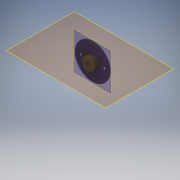
# Autodesk Inventor part: capot_inf
Saved by Autodesk Inventor 2018 (Build 220112000, 112)
## iProperties
Created: 2017-10-08
Part Number: capot_inf
Material: Iron, Cast
Document SubType Name: Modeling
Designer: liamg
Density: 7.15 g/cm^3
Appearance: Iron Gray
Author: liamg
Autodesk Inventor part; units mm, degrees
ref_plane "YZ Plane" through (0, 0, 0) normal (1, 0, 0) x (0, 1, 0)
ref_plane "XY Plane" through (0, 0, 0) normal (0, 0, 1) x (1, 0, 0)
ref_plane "Work Plane1" through (-71.4709, -34.2956, -57.6282) normal (0, 0, -1) x (-1, 0, 0)
sketch "Sketch1" plane through (-71.4709, -34.2956, -57.6282) normal (0, 0, -1) x (-1, 0, 0)
  circle A0 centre (0, 0) radius 17.93 projected
  point P0 (-71.4709, 34.2956)
extrude "Extrusion1" add sketch "Sketch1" along normal blind 0.8
sketch "Sketch2" plane through (-71.4709, -34.2956, -57.6282) normal (0, 0, 1) x (1, 0, 0)
  circle A0 centre (0, 0) radius 12.175 construction
  circle A1 centre (12.175, 0) radius 1.415
  circle A2 centre (-12.175, 0) radius 1.415
  point P0 (71.4709, 34.2956)
  dimension "d2" = 24.35
  dimension "d3" = 2.83
  dimension "d4" = 2.83
  constraints: 3 centre point, 2 point on circle
  measures "d2" diameter of A0
  measures "d3" diameter of A1
  measures "d4" diameter of A2
extrude "Extrusion2" cut sketch "Sketch2" against normal blind 0.8
sketch "Sketch3" plane through (-71.4709, -34.2956, -57.6282) normal (0, 0, 1) x (1, 0, 0)
  circle A0 centre (0, 0) radius 6.5
  point P0 (71.4709, 34.2956)
  dimension "d7" = 13
  constraints: 1 centre point
  measures "d7" diameter of A0
extrude "Extrusion3" add sketch "Sketch3" along normal blind 4.5
fillet "Fillet1" radius 0.508 1 edges at (-77.9709, -34.2956, -53.1282)
sketch "Sketch4" plane through (-71.4709, -34.2956, -53.1282) normal (0, 0, 1) x (1, 0, 0)
  circle A0 centre (0, 0) radius 1.6
  point P0 (71.4709, 34.2956)
  dimension "d11" = 3.2
  constraints: 1 centre point
  measures "d11" diameter of A0
extrude "Extrusion4" cut sketch "Sketch4" against normal blind 19.2875
body "Solid1"
